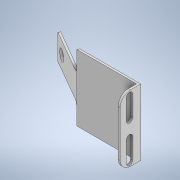
# Autodesk Inventor part: Lampenhalterung 2,0
Saved by Autodesk Inventor 2021.3 (Build 253353000, 353)
## iProperties
Created: 2021-10-12
Part Number: Lampenhalterung 2,0
Material: Generisch
Document SubType Name: Modeling
Designer: bhelg
Density: 1 g/cm^3
Appearance: Vorgabe
Author: bhelg
Autodesk Inventor part; units mm, degrees
ref_plane "YZ Plane" through (0, 0, 0) normal (1, 0, 0) x (0, 1, 0)
ref_plane "XZ Plane" through (0, 0, 0) normal (0, 1, 0) x (-1, 0, 0)
ref_plane "XY Plane" through (0, 0, 0) normal (0, 0, 1) x (1, 0, 0)
sketch "Skizze1" plane through (0, 0, 0) normal (0, 1, 0) x (-1, 0, 0)
  line L0 (0, 0) -> (0, -2)
  line L1 (0, -2) -> (60, -2)
  line L2 (60, -2) -> (103.3013, -27)
  line L3 (103.3013, -27) -> (104.3013, -25.2679)
  line L4 (0, 0) -> (60.5359, 0)
  line L5 (104.3013, -25.2679) -> (60.5359, 0)
  dimension "d0" = 2
  dimension "d1" = 60
  dimension "d2" = 50
  dimension "d3" = 150
  dimension "d4" = 2
  dimension "d42" = 0
  constraints: 12 end point, 2 perpendicular, 1 horizontal, 1 vertical
  measures "d0" distance of L0.start L0.end
  measures "d1" distance of L0.end L1.end
  measures "d2" distance of L1.end L2.end
  measures "d3" angle of L1 L2
  measures "d4" distance of L2.end L3.end
  measures "d42" angle of L2 L5
extrude "Extrusion1" add sketch "Skizze1" along normal blind 65
sketch "Skizze2" plane through (-60.5359, 0, 0) normal (0, 0, 1) x (1, 0, 0)
  line L0 (60.5359, 0) -> (0.5359, 0) projected
  line L1 (60.5359, 0) -> (58.5359, 0)
  line L2 (58.5359, 0) -> (58.5359, 65)
  line L3 (58.5359, 65) -> (60.5359, 65)
  line L4 (60.5359, 65) -> (60.5359, 0)
  point P0 (58.5359, 0)
  dimension "d8" = 2
  dimension "d9" = 65
  constraints: 8 end point, 2 parallel, 1 horizontal, 1 perpendicular
  measures "d8" distance of L2.end L3.end
  measures "d9" distance of L1.end L2.end
extrude "Extrusion2" add sketch "Skizze2" along normal blind 18
sketch "Skizze3" plane through (-2, 0, 0) normal (-1, 0, 0) x (0, 0, 1)
  line L0 (0, 0) -> (18, 0) projected
  line L1 (18, 65) -> (18, 0) projected
  line L2 (9, 24.5) -> (9, 4.5) construction
  line L3 (5.9, 24.5) -> (5.9, 4.5)
  line L4 (12.1, 4.5) -> (12.1, 24.5)
  arc A0 (12.1, 24.5) -> (5.9, 24.5) centre (9, 24.5) ccw
  arc A1 (5.9, 4.5) -> (12.1, 4.5) centre (9, 4.5) ccw
  line L5 (9, 60.5) -> (9, 40.5) construction
  line L6 (5.9, 60.5) -> (5.9, 40.5)
  line L7 (12.1, 40.5) -> (12.1, 60.5)
  arc A2 (12.1, 60.5) -> (5.9, 60.5) centre (9, 60.5) ccw
  arc A3 (5.9, 40.5) -> (12.1, 40.5) centre (9, 40.5) ccw
  line L8 (0, 0) -> (0, 65) projected
  point P0 (9, 14.5)
  point P1 (9, 50.5)
  dimension "d12" = 36
  dimension "d32" = 6.2
  dimension "d34" = 20
  dimension "d35" = 14.5
  dimension "d36" = 6.2
  dimension "d37" = 20
  dimension "d43" = 9
  dimension "d44" = 18
  constraints: 16 end point, 8 point on circle, 8 tangent, 4 centre point, 3 equal length, 2 midpoint, 1 point on line, 1 vertical
  measures "d12" distance of L5.start L2.start
  measures "d32" distance between parallel lines of L3 L4
  measures "d34" distance of L2.end L2.start
  measures "d35" distance from line of point (9, 14.5) L0
  measures "d36" distance between parallel lines of L6 L7
  measures "d37" distance of L5.end L5.start
  measures "d43" distance from line of L8 L2.end
  measures "d44" distance between parallel lines of L8 L1
sketch "Skizze4" plane through (-60.5359, 0, 0) normal (-0.5, 0, 0.8660254) x (0.8660254, 0, 0.5)
  line L0 (-50.5359, 0) -> (0, 0) projected
  line L1 (-50.5359, 0) -> (-50.5359, 65) projected
  point P0 (52.4256, 0)
  point P1 (-40.5359, 32.5)
  dimension "d23" = 32.5
  dimension "d24" = 10
  measures "d23" distance from line of point (-40.536, 32.5) L0
  measures "d24" distance from line of L1 point (-40.536, 32.5)
hole "Bohrung2" at (-95.641, 32.5, -20.2679) direction (0.5, 0, -0.8660254) diameter 10.4 end through all
extrude "Extrusion3" cut sketch "Skizze3" against normal blind 10
fillet "Rundung1" radius 10 4 edges at (-103.8013, 65, -26.134) (-103.8013, 0, -26.134) (-1, 0, 18) (-1, 65, 18)
sketch "Skizze6" plane through (-60.5359, 0, 0) normal (-0.5, 0, 0.8660254) x (0.8660254, 0, 0.5)
  line L0 (0, 0) -> (0, 65) projected
  line L1 (0, 0) -> (-50.536, 0)
  line L2 (-50.536, 0) -> (-50.536, 20)
  line L3 (-50.536, 20) -> (0, 20)
  line L4 (0, 20) -> (0, 0)
  line L5 (-40.5359, 65) -> (0, 65) projected
  line L6 (0, 65) -> (-50.536, 65)
  line L7 (-50.536, 65) -> (-50.536, 45)
  line L8 (-50.536, 45) -> (0, 45)
  line L9 (0, 45) -> (0, 65)
  point P0 (52.4256, 0)
  point P1 (0, 45)
  point P2 (0, 20)
  dimension "d46" = 50.536
  dimension "d47" = 20
  dimension "d48" = 50.536
  dimension "d49" = 20
  constraints: 16 end point, 4 parallel, 2 horizontal, 2 perpendicular
  measures "d46" distance of L2.end L3.end
  measures "d47" distance of L1.end L2.end
  measures "d48" distance of L8.end L7.end
  measures "d49" distance of L7.end L6.end
extrude "Extrusion4" cut sketch "Skizze6" against normal blind 10
fillet "Rundung2" radius 4 2 edges at (-59.9585, 20, -1) (-59.9585, 45, -1)
equation "\"d36\" = d32"
equation "\"d37\" = d34"
equation "\"d43\" = 0.5 * d44"
